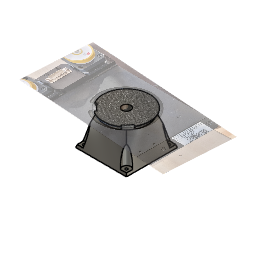
stage-post v3 (Autodesk Fusion 360 design; units mm, degrees)
Autodesk Fusion 360 part; units mm, degrees
note: some values were not read from the file. Chosen so that the rebuilt part matches the saved one: which face or edge a step refers to.
sketch "Sketch1" plane through (0, 0, 0) normal (0, 0, 1) x (1, 0, 0)
  line L0 (60, 60) -> (-60, 60)
  line L1 (-60, 60) -> (-60, -60)
  line L2 (-60, -60) -> (60, -60)
  line L3 (60, -60) -> (60, 60)
  line L4 (60, 60) -> (-60, -60) construction
  line L5 (-60, 60) -> (60, -60) construction
  dimension "d1" = 120
  dimension "d2" = 120
  constraint horizontal L0
  constraint perpendicular L0 L1
  constraint parallel L0 L2
  constraint parallel L1 L3
  constraint coincident L4 origin
  constraint coincident L5 origin
  measures "d1" distance of L1.end L2.end
  measures "d2" distance of L0.end L1.end
ref_plane "WorkPlane1" through (0, 0, 80) normal (0, 0, 1) x (1, 0, 0)
sketch "Sketch2" plane through (0, 0, 80) normal (0, 0, 1) x (1, 0, 0)
  circle A0 centre (0, 0) radius 55
  dimension "d4" = 110
  constraint coincident A0.centre origin
  measures "d4" diameter of A0
loft "Loft1" add profiles "Sketch1", "Sketch2" section 1 section 2 makes body 1
sketch "Sketch3" plane through (0, 0, 0) normal (0, 1, 0) x (1, 0, 0)
  line L0 (60, 0) -> (38.8909, -80)
  line L1 (38.8909, -80) -> (55, -80)
  line L2 (38.8909, -80) -> (60, 0)
  line L3 (55, -80) -> (50, -71.3397)
  line L4 (55, -80) -> (60, -80) construction
  line L5 (50, -71.3397) -> (70.5852, -71.3397)
  line L6 (70.5852, -71.3397) -> (70.5852, -80)
  line L7 (70.5852, -80) -> (55, -80)
  dimension "d5" = 120
  dimension "d6" = 10
  constraint horizontal L4
  constraint coincident L1.end L3.start
  constraint horizontal L5
  constraint perpendicular L5 L6
  measures "d5" angle of L3 L4
  measures "d6" distance of L1.end L3.end
revolve "Revolve1" cut sketch "Sketch3" angle 360 about axis through (0, 0, 1.75) along (0, 0, 1) bodies 1
split "Split1" by plane through (0, 0, 71.3397) normal (0, 0, 1) bodies 1 makes body 2 at (-1.9798, 15.6107, 80)
delete_body "RemoveBody1" bodies 1
loft "Loft2" add profiles "Sketch1" section 1 section 2 face at (-13.5518, -2.484, 71.3397) on bodies 2 bodies 2
extrude "Extrude1" add 1 faces at (-1.9798, 15.6107, 80) along direction (0, 0, 1) blind 1 on bodies 2 bodies 2
sketch "Sketch4" plane through (0, 0, 0) normal (0, 0, 1) x (1, 0, 0)
  circle A0 centre (0, 0) radius 3
  circle A1 centre (-50, -50) radius 3
  circle A2 centre (-25, -50) radius 3
  circle A3 centre (0, -50) radius 3
  circle A4 centre (25, -50) radius 3
  circle A5 centre (50, -50) radius 3
  circle A6 centre (-50, -25) radius 3
  circle A7 centre (-25, -25) radius 3
  circle A8 centre (0, -25) radius 3
  circle A9 centre (25, -25) radius 3
  circle A10 centre (50, -25) radius 3
  circle A11 centre (-50, 0) radius 3
  circle A12 centre (-25, 0) radius 3
  circle A13 centre (25, 0) radius 3
  circle A14 centre (50, 0) radius 3
  circle A15 centre (-50, 25) radius 3
  circle A16 centre (-25, 25) radius 3
  circle A17 centre (0, 25) radius 3
  circle A18 centre (25, 25) radius 3
  circle A19 centre (50, 25) radius 3
  circle A20 centre (-50, 50) radius 3
  circle A21 centre (-25, 50) radius 3
  circle A22 centre (0, 50) radius 3
  circle A23 centre (25, 50) radius 3
  circle A24 centre (50, 50) radius 3
  dimension "d10" = 6
  dimension "d13" = 0
  dimension "d14" = 0
  dimension "d17" = 25
  dimension "d18" = 25
  constraint coincident A0.centre origin
  measures "d10" diameter of A0
extrude "Extrude2" cut sketch "Sketch4" along normal blind 90 contours A0 | A1 | A5 | A20 | A24 bodies 2
sketch "Sketch5" plane through (0, 0, 81) normal (0, 0, 1) x (-1, 0, 0)
  circle A0 centre (0, 0) radius 3
  circle A1 centre (0, 0) radius 55
  circle A2 centre (0, 0) radius 10
  dimension "d21" = 20
  constraint concentric A0 A2
  measures "d21" diameter of A2
extrude "Extrude3" cut sketch "Sketch5" against normal blind 75 contours A2 bodies 2
sketch "Sketch7" plane through (0, 0, 6) normal (0, 0, 1) x (-1, 0, 0)
  circle A0 centre (0, 0) radius 3
  circle A1 centre (0, 0) radius 10
  spline S0 degree 3 poles (52.1213, -52.1213) (51.8932, -52.3495) (51.6303, -52.5388) (51.1885, -52.7599) (51.0108, -52.8322) (50.6972, -52.9203) (50.5789, -52.9462) (50.3541, -52.9808) (50.2525, -52.991) (50.0263, -53.0026) (49.9065, -53.0007) (49.5614, -52.9769) (49.3566, -52.9357) (48.7305, -52.7587) (48.3225, -52.5288) (47.3017, -51.6027) (46.9363, -50.6984) (47.0434, -49.3276) (47.1727, -48.9007) (47.5098, -48.3113) (47.6654, -48.0919) (47.8787, -47.8787) knots -1.701663 -1.701663 -1.701663 -1.701663 -1.546732 -1.546732 -1.46381 -1.46381 -1.416501 -1.416501 -1.376691 -1.376691 -1.326354 -1.326354 -1.222013 -1.222013 -0.94765 -0.94765 -0.393897 -0.393897 -0.133141 -0.133141 0 0 0 0
  spline S1 degree 3 poles (47.8787, -47.8787) (48.1104, -47.6469) (48.35, -47.4826) (48.7793, -47.2487) (48.9906, -47.1674) (49.9598, -46.8953) (50.7582, -47.0004) (51.8533, -47.591) (52.2256, -47.9268) (52.6374, -48.5494) (52.8209, -48.8809) (52.9596, -49.4839) (52.988, -49.6646) (53.0018, -49.9738) (53.0011, -50.0874) (52.9859, -50.3073) (52.9738, -50.4092) (52.9333, -50.6429) (52.9026, -50.7686) (52.8019, -51.0934) (52.7216, -51.2742) (52.5003, -51.6829) (52.3263, -51.9164) (52.1213, -52.1213) knots -2.547832 -2.547832 -2.547832 -2.547832 -2.331835 -2.331835 -2.11682 -2.11682 -1.281775 -1.281775 -0.743294 -0.743294 -0.480328 -0.480328 -0.388187 -0.388187 -0.338971 -0.338971 -0.297158 -0.297158 -0.243576 -0.243576 -0.151478 -0.151478 0 0 0 0
  circle A2 centre (50, -50) radius 3
  spline S2 degree 3 poles (-52.1213, -52.1213) (-52.3495, -51.8932) (-52.5388, -51.6303) (-52.7599, -51.1885) (-52.8322, -51.0108) (-52.9203, -50.6972) (-52.9462, -50.5789) (-52.9808, -50.3541) (-52.991, -50.2525) (-53.0026, -50.0263) (-53.0007, -49.9065) (-52.9769, -49.5614) (-52.9357, -49.3566) (-52.7587, -48.7305) (-52.5288, -48.3225) (-51.6027, -47.3017) (-50.6984, -46.9363) (-49.3276, -47.0434) (-48.9007, -47.1727) (-48.3113, -47.5098) (-48.0919, -47.6654) (-47.8787, -47.8787) knots -1.701663 -1.701663 -1.701663 -1.701663 -1.546732 -1.546732 -1.46381 -1.46381 -1.416501 -1.416501 -1.376691 -1.376691 -1.326354 -1.326354 -1.222013 -1.222013 -0.94765 -0.94765 -0.393897 -0.393897 -0.133141 -0.133141 0 0 0 0
  spline S3 degree 3 poles (-47.8787, -47.8787) (-47.6469, -48.1104) (-47.4826, -48.35) (-47.2487, -48.7793) (-47.1674, -48.9906) (-46.8953, -49.9598) (-47.0004, -50.7582) (-47.591, -51.8533) (-47.9268, -52.2256) (-48.5494, -52.6374) (-48.8809, -52.8209) (-49.4839, -52.9596) (-49.6646, -52.988) (-49.9738, -53.0018) (-50.0874, -53.0011) (-50.3073, -52.9859) (-50.4092, -52.9738) (-50.6429, -52.9333) (-50.7686, -52.9026) (-51.0934, -52.8019) (-51.2742, -52.7216) (-51.6829, -52.5003) (-51.9164, -52.3263) (-52.1213, -52.1213) knots -2.547832 -2.547832 -2.547832 -2.547832 -2.331835 -2.331835 -2.11682 -2.11682 -1.281775 -1.281775 -0.743294 -0.743294 -0.480328 -0.480328 -0.388187 -0.388187 -0.338971 -0.338971 -0.297158 -0.297158 -0.243576 -0.243576 -0.151478 -0.151478 0 0 0 0
  circle A3 centre (-50, -50) radius 3
  spline S4 degree 3 poles (-47.8787, 47.8787) (-48.1104, 47.6469) (-48.35, 47.4826) (-48.7793, 47.2487) (-48.9906, 47.1674) (-49.9598, 46.8953) (-50.7582, 47.0004) (-51.8533, 47.591) (-52.2256, 47.9268) (-52.6374, 48.5494) (-52.8209, 48.8809) (-52.9596, 49.4839) (-52.988, 49.6646) (-53.0018, 49.9738) (-53.0011, 50.0874) (-52.9859, 50.3073) (-52.9738, 50.4092) (-52.9333, 50.6429) (-52.9026, 50.7686) (-52.8019, 51.0934) (-52.7216, 51.2742) (-52.5003, 51.6829) (-52.3263, 51.9164) (-52.1213, 52.1213) knots -2.547832 -2.547832 -2.547832 -2.547832 -2.331835 -2.331835 -2.11682 -2.11682 -1.281775 -1.281775 -0.743294 -0.743294 -0.480328 -0.480328 -0.388187 -0.388187 -0.338971 -0.338971 -0.297158 -0.297158 -0.243576 -0.243576 -0.151478 -0.151478 0 0 0 0
  spline S5 degree 3 poles (-52.1213, 52.1213) (-51.8932, 52.3495) (-51.6303, 52.5388) (-51.1885, 52.7599) (-51.0108, 52.8322) (-50.6972, 52.9203) (-50.5789, 52.9462) (-50.3541, 52.9808) (-50.2525, 52.991) (-50.0263, 53.0026) (-49.9065, 53.0007) (-49.5614, 52.9769) (-49.3566, 52.9357) (-48.7305, 52.7587) (-48.3225, 52.5288) (-47.3017, 51.6027) (-46.9363, 50.6984) (-47.0434, 49.3276) (-47.1727, 48.9007) (-47.5098, 48.3113) (-47.6654, 48.0919) (-47.8787, 47.8787) knots -1.701663 -1.701663 -1.701663 -1.701663 -1.546732 -1.546732 -1.46381 -1.46381 -1.416501 -1.416501 -1.376691 -1.376691 -1.326354 -1.326354 -1.222013 -1.222013 -0.94765 -0.94765 -0.393897 -0.393897 -0.133141 -0.133141 0 0 0 0
  circle A4 centre (-50, 50) radius 3
  spline S6 degree 3 poles (52.1213, 52.1213) (52.3495, 51.8932) (52.5388, 51.6303) (52.7599, 51.1885) (52.8322, 51.0108) (52.9203, 50.6972) (52.9462, 50.5789) (52.9808, 50.3541) (52.991, 50.2525) (53.0026, 50.0263) (53.0007, 49.9065) (52.9769, 49.5614) (52.9357, 49.3566) (52.7587, 48.7305) (52.5288, 48.3225) (51.6027, 47.3017) (50.6984, 46.9363) (49.3276, 47.0434) (48.9007, 47.1727) (48.3113, 47.5098) (48.0919, 47.6654) (47.8787, 47.8787) knots -1.701663 -1.701663 -1.701663 -1.701663 -1.546732 -1.546732 -1.46381 -1.46381 -1.416501 -1.416501 -1.376691 -1.376691 -1.326354 -1.326354 -1.222013 -1.222013 -0.94765 -0.94765 -0.393897 -0.393897 -0.133141 -0.133141 0 0 0 0
  spline S7 degree 3 poles (47.8787, 47.8787) (47.6469, 48.1104) (47.4826, 48.35) (47.2487, 48.7793) (47.1674, 48.9906) (46.8953, 49.9598) (47.0004, 50.7582) (47.591, 51.8533) (47.9268, 52.2256) (48.5494, 52.6374) (48.8809, 52.8209) (49.4839, 52.9596) (49.6646, 52.988) (49.9738, 53.0018) (50.0874, 53.0011) (50.3073, 52.9859) (50.4092, 52.9738) (50.6429, 52.9333) (50.7686, 52.9026) (51.0934, 52.8019) (51.2742, 52.7216) (51.6829, 52.5003) (51.9164, 52.3263) (52.1213, 52.1213) knots -2.547832 -2.547832 -2.547832 -2.547832 -2.331835 -2.331835 -2.11682 -2.11682 -1.281775 -1.281775 -0.743294 -0.743294 -0.480328 -0.480328 -0.388187 -0.388187 -0.338971 -0.338971 -0.297158 -0.297158 -0.243576 -0.243576 -0.151478 -0.151478 0 0 0 0
  circle A5 centre (50, 50) radius 3
  circle A6 centre (-50, 50) radius 10
  circle A7 centre (0, 0) radius 3
  circle A8 centre (-50, -50) radius 3
  circle A9 centre (50, -50) radius 3
  circle A10 centre (50, 50) radius 3
  circle A11 centre (-50, 50) radius 3
  line L0 (-60, -60) -> (-60, 60)
  line L1 (-60, 60) -> (60, 60)
  line L2 (60, 60) -> (60, -60)
  line L3 (60, -60) -> (-60, -60)
  circle A12 centre (50, 50) radius 10
  circle A13 centre (-50, -50) radius 10
  circle A14 centre (50, -50) radius 10
  dimension "d24" = 20
  dimension "d27" = 100
  dimension "d28" = -100
  constraint concentric A4 A6
  measures "d24" diameter of A6
extrude "Extrude4" cut sketch "Sketch7" along normal blind 54.954 contours S0 S1 A2 A9 | S2 S3 A3 A8 | S4 S5 A4 A11 | S6 S7 A5 A10 | A6 | A6 L0 L1 | L1 L2 A12 | A12 | L0 L3 A13 | A13 | A14 | L2 L3 A14 bodies 2
sketch "Sketch8" plane through (0, 0, 81) normal (0, 0, 1) x (-1, 0, 0)
  circle A0 centre (0, 0) radius 10
  circle A1 centre (0, 0) radius 55
sketch "Sketch9" plane through (0, 0, 81) normal (0, 0, 1) x (-1, 0, 0)
  line L0 (0, 0) -> (-86.1031, 49.7116)
  line L1 (0, 0) -> (0, 92.4891)
  circle A0 centre (0, 0) radius 55
  line L2 (0, 0) -> (100, 0) construction
  line L3 (0, 0) -> (-57.0134, 81.4236)
  circle A1 centre (0, 0) radius 50
  circle A2 centre (0, 0) radius 55
  line L4 (0, 0) -> (86.1031, 49.7116)
  line L5 (0, 0) -> (57.0134, 81.4236)
  dimension "d34" = 60
  dimension "d41" = 35
  dimension "d42" = 100
  dimension "d43" = 110
  constraint coincident L0.start L1.start
  constraint vertical L1
  constraint symmetric L0.start L1 A0.centre
  constraint horizontal L2
  constraint concentric A0 A1
  constraint symmetric L0.end L1 L4.end
  constraint symmetric L1 L0.start A0.centre
  constraint symmetric L1 L3.end L5.end
  measures "d34" angle of L0 L1
  measures "d41" angle of L1 L3
  measures "d42" diameter of A1
  measures "d43" diameter of A2
extrude "Extrude6" cut sketch "Sketch9" against normal blind 9.6655 contours L0 A0 L3 A1 A2 | A0 A1 A2 L4 L5 bodies 2
equation "d5 = 180 deg - 45 deg - 15 deg"
